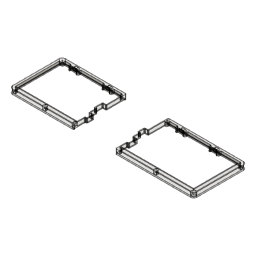
KBO-5000-Case-Redesign-Body (Autodesk Fusion 360 design; units mm, degrees)
Autodesk Fusion 360 part; units mm, degrees
(part 1 of 2)
other "Base Mesh Feature1"
sketch "Left-Main" plane through (0, 0, 0) normal (0, 0, 1) x (1, 0, 0)
  line L0 (-242, 0) -> (-78.0749, 0)
  line L1 (-250, 8) -> (-250, 135.063)
  line L2 (-242, 143.063) -> (-78.075, 143.063)
  line L3 (-76.075, 141.063) -> (-76.075, 90.2)
  line L4 (-78.075, 88.2) -> (-83.6, 88.2)
  line L5 (-85.6, 86.2) -> (-85.6, 71.15)
  line L6 (-83.6, 69.15) -> (-82.837, 69.15)
  line L7 (-80.837, 67.15) -> (-80.837, 52.1)
  line L8 (-78.837, 50.1) -> (-73.312, 50.1)
  line L9 (-71.312, 48.1) -> (-71.312, 33.05)
  line L10 (-73.312, 31.05) -> (-74.0741, 31.05)
  line L11 (-76.0741, 29.0501) -> (-76.0749, 1.9999)
  arc A0 (-242, 143.063) -> (-250, 135.063) centre (-242, 135.063) ccw
  arc A1 (-250, 8) -> (-242, 0) centre (-242, 8) ccw
  line L12 (-78.074, 32.05) -> (-78.0749, 2)
  line L13 (-242, 2) -> (-78.0749, 2)
  arc A2 (-248, 8) -> (-242, 2) centre (-242, 8) ccw
  line L14 (-248, 8) -> (-248, 135.063)
  arc A3 (-242, 141.063) -> (-248, 135.063) centre (-242, 135.063) ccw
  line L15 (-242, 141.063) -> (-78.075, 141.063)
  line L16 (-78.075, 141.063) -> (-78.075, 91.2)
  line L17 (-79.075, 90.2) -> (-86.6, 90.2)
  line L18 (-87.6, 89.2) -> (-87.6, 68.15)
  line L19 (-86.6, 67.15) -> (-83.837, 67.15)
  line L20 (-82.837, 66.15) -> (-82.837, 49.1)
  line L21 (-81.837, 48.1) -> (-74.312, 48.1)
  line L22 (-73.312, 47.1) -> (-73.312, 34.05)
  line L23 (-74.312, 33.05) -> (-77.074, 33.05)
  line L24 (-238.001, 131.063) -> (-237.9999, 12.005)
  line L25 (-78.075, 141.063) -> (-78.075, 131.063)
  arc A4 (-76.075, 141.063) -> (-78.075, 143.063) centre (-78.075, 141.063) ccw
  arc A5 (-78.0749, 0) -> (-76.0749, 1.9999) centre (-78.0749, 2) ccw
  arc A6 (-73.312, 31.05) -> (-71.312, 33.05) centre (-73.312, 33.05) ccw
  arc A7 (-71.312, 48.1) -> (-73.312, 50.1) centre (-73.312, 48.1) ccw
  arc A8 (-80.837, 52.1) -> (-78.837, 50.1) centre (-78.837, 52.1) ccw
  arc A9 (-80.837, 67.15) -> (-82.837, 69.15) centre (-82.837, 67.15) ccw
  arc A10 (-85.6, 71.15) -> (-83.6, 69.15) centre (-83.6, 71.15) ccw
  arc A11 (-83.6, 88.2) -> (-85.6, 86.2) centre (-83.6, 86.2) ccw
  arc A12 (-78.075, 88.2) -> (-76.075, 90.2) centre (-78.075, 90.2) ccw
  arc A13 (-79.075, 90.2) -> (-78.075, 91.2) centre (-79.075, 91.2) ccw
  arc A14 (-86.6, 90.2) -> (-87.6, 89.2) centre (-86.6, 89.2) ccw
  arc A15 (-87.6, 68.15) -> (-86.6, 67.15) centre (-86.6, 68.15) ccw
  arc A16 (-82.837, 66.15) -> (-83.837, 67.15) centre (-83.837, 66.15) ccw
  arc A17 (-82.837, 49.1) -> (-81.837, 48.1) centre (-81.837, 49.1) ccw
  arc A18 (-73.312, 47.1) -> (-74.312, 48.1) centre (-74.312, 47.1) ccw
  arc A19 (-74.312, 33.05) -> (-73.312, 34.05) centre (-74.312, 34.05) ccw
  arc A20 (-77.074, 33.05) -> (-78.074, 32.05) centre (-77.074, 32.05) ccw
  arc A21 (-74.0741, 31.05) -> (-76.0741, 29.0501) centre (-74.0741, 29.05) ccw
  line L26 (-237.9999, 12.005) -> (-78.0746, 11.9998)
  line L27 (-238.001, 131.063) -> (-78.075, 131.063)
  point P0 (-250, 0)
  point P1 (-76.075, 0)
  point P2 (-250, 143.063)
  point P3 (-76.075, 143.063)
  point P4 (-76.075, 88.2)
  point P5 (-85.6, 88.2)
  point P6 (-85.6, 69.15)
  point P7 (-80.837, 69.15)
  point P8 (-80.837, 50.1)
  point P9 (-71.312, 50.1)
  point P10 (-71.312, 31.05)
  point P11 (-76.074, 31.05)
  point P12 (-78.075, 131.063)
  dimension "d1" = 173.925
  dimension "d2" = 143.063
  dimension "d3" = 173.925
  dimension "d4" = 54.863
  dimension "d5" = 9.525
  dimension "d6" = 19.05
  dimension "d7" = 4.763
  dimension "d8" = 19.05
  dimension "d9" = 9.525
  dimension "d10" = 19.05
  dimension "d11" = 4.762
  dimension "d12" = 31.05
  dimension "d13" = 8
  dimension "d14" = 8
  dimension "d31" = 10
  dimension "d34" = 2
  dimension "d35" = 2
  dimension "d36" = 2
  dimension "d37" = 2
  dimension "d38" = 2
  dimension "d39" = 2
  dimension "d40" = 2
  dimension "d41" = 2
  dimension "d42" = 2
  dimension "d43" = 1
  dimension "d44" = 2
  dimension "d82" = 119.058
  constraint horizontal L0
  constraint perpendicular L0 L1
  constraint perpendicular L1 L2
  constraint perpendicular L2 L3
  constraint perpendicular L3 L4
  constraint perpendicular L4 L5
  constraint perpendicular L5 L6
  constraint perpendicular L6 L7
  constraint perpendicular L7 L8
  constraint perpendicular L8 L9
  constraint perpendicular L9 L10
  constraint coincident P2 L1
  constraint coincident P2 L2
  constraint tangent L1 A0
  constraint tangent L2 A0
  constraint coincident P0 L0
  constraint coincident P0 L1
  constraint tangent L0 A1
  constraint tangent L1 A1
  constraint concentric A1 A2
  constraint concentric A0 A3
  constraint tangent A3 L15
  constraint tangent L13 A2
  constraint tangent A2 L14
  constraint tangent L14 A3
  constraint coincident P12 L25.end
  constraint coincident P3 L2
  constraint coincident P3 L3
  constraint tangent L2 A4
  constraint tangent L3 A4
  constraint coincident P1 L0
  constraint coincident P1 L11
  constraint tangent L0 A5
  constraint tangent L11 A5
  constraint coincident P10 L9
  constraint coincident P10 L10
  constraint tangent L9 A6
  constraint tangent L10 A6
  constraint coincident P9 L8
  constraint coincident P9 L9
  constraint tangent L8 A7
  constraint tangent L9 A7
  constraint coincident P8 L7
  constraint coincident P8 L8
  constraint tangent L7 A8
  constraint tangent L8 A8
  constraint coincident P7 L6
  constraint coincident P7 L7
  constraint tangent L6 A9
  constraint tangent L7 A9
  constraint coincident P6 L5
  constraint coincident P6 L6
  constraint tangent L5 A10
  constraint tangent L6 A10
  constraint coincident P5 L4
  constraint coincident P5 L5
  constraint tangent L4 A11
  constraint tangent L5 A11
  constraint coincident P4 L3
  constraint coincident P4 L4
  constraint tangent L3 A12
  constraint tangent L4 A12
  constraint tangent L16 A13
  constraint tangent L17 A13
  constraint tangent L17 A14
  constraint tangent L18 A14
  constraint equal A13 A14
  constraint tangent L18 A15
  constraint tangent L19 A15
  constraint equal A13 A15
  constraint tangent L19 A16
  constraint tangent L20 A16
  constraint equal A13 A16
  constraint tangent L20 A17
  constraint tangent L21 A17
  constraint equal A13 A17
  constraint tangent L21 A18
  constraint tangent L22 A18
  constraint equal A13 A18
  constraint tangent L22 A19
  constraint tangent L23 A19
  constraint equal A13 A19
  constraint tangent L12 A20
  constraint tangent L23 A20
  constraint equal A13 A20
  constraint coincident P11 L10
  constraint coincident P11 L11
  constraint tangent L10 A21
  constraint tangent L11 A21
  constraint coincident L12 L26.end
  constraint perpendicular L12 L26
  constraint perpendicular L25 L27
  measures "d1" distance of P0 P1
  measures "d2" distance of P0 P2
  measures "d3" distance of P2 P3
  measures "d4" distance of P3 P4
  measures "d5" distance of P4 P5
  measures "d6" distance of P5 P6
  measures "d7" distance of P6 P7
  measures "d8" distance of P7 P8
  measures "d9" distance of P8 P9
  measures "d10" distance of P9 P10
  measures "d11" distance of P10 P11
  measures "d12" distance of L0 L10
  measures "d13" radius of A0
  measures "d14" radius of A1
  measures "d31" distance of L15.end P12
  measures "d34" radius of A4
  measures "d35" radius of A5
  measures "d36" radius of A6
  measures "d37" radius of A7
  measures "d38" radius of A8
  measures "d39" radius of A9
  measures "d40" radius of A10
  measures "d41" radius of A11
  measures "d42" radius of A12
  measures "d43" radius of A13
  measures "d44" radius of A21
  measures "d82" vertical distance of L24.start L24.end
sketch "Left-Bottom" plane through (0, 0, 0) normal (0, 0, 1) x (1, 0, 0)
  line L0 (-76.0749, 3.75) -> (-76.0749, 1.9999)
  line L1 (-78.0749, 0) -> (-242, 0)
  line L2 (-76.0749, 3.75) -> (-242, 3.7553)
  line L3 (-78.075, 143.063) -> (-242, 143.063)
  line L4 (-76.075, 141.063) -> (-76.075, 139.313)
  line L5 (-76.075, 139.313) -> (-242, 139.313)
  line L6 (-250, 135.063) -> (-250, 8)
  line L7 (-246.25, 135.063) -> (-246.2499, 8.0053)
  arc A0 (-250, 8) -> (-242, 0) centre (-242, 8) ccw
  arc A1 (-242, 143.063) -> (-250, 135.063) centre (-242, 135.063) ccw
  arc A2 (-242, 139.313) -> (-246.25, 135.063) centre (-242, 135.063) ccw
  arc A3 (-246.2499, 8.0053) -> (-242, 3.7553) centre (-241.9999, 8.0053) ccw
  arc A4 (-76.075, 141.063) -> (-78.075, 143.063) centre (-78.075, 141.063) ccw
  arc A5 (-78.0749, 0) -> (-76.0749, 1.9999) centre (-78.0749, 2) ccw
  circle A6 centre (-80.0748, 135.0624) radius 2.9
  circle A7 centre (-80.0748, 135.0624) radius 1.2
  circle A8 centre (-80.0749, 8) radius 2.9
  circle A9 centre (-80.0749, 8) radius 1.2
  circle A10 centre (-108.9375, 135.0625) radius 1.2
  circle A11 centre (-128.9375, 135.0625) radius 1.2
  circle A12 centre (-199.425, 135.0625) radius 1.2
  circle A13 centre (-219.425, 135.0625) radius 1.2
  circle A14 centre (-241.4142, 134.4767) radius 1.2
  circle A15 centre (-241.4142, 8.5857) radius 1.2
  circle A16 centre (-160.0375, 8) radius 1.2
  circle A17 centre (-241.4142, 134.4767) radius 2.9
  circle A18 centre (-241.4142, 8.5857) radius 2.9
  circle A19 centre (-160.0375, 8) radius 2.9
  line L8 (-126.938, 132.063) -> (-126.938, 133.063)
  line L9 (-125.938, 134.063) -> (-111.938, 134.063)
  line L10 (-110.938, 133.063) -> (-110.938, 132.063)
  arc A20 (-125.938, 134.063) -> (-126.938, 133.063) centre (-125.938, 133.063) ccw
  arc A21 (-110.938, 133.063) -> (-111.938, 134.063) centre (-111.938, 133.063) ccw
  line L11 (-109.938, 131.063) -> (-108.938, 131.063)
  line L12 (-127.938, 131.063) -> (-128.938, 131.063)
  arc A22 (-110.938, 132.063) -> (-109.938, 131.063) centre (-109.938, 132.063) ccw
  arc A23 (-127.938, 131.063) -> (-126.938, 132.063) centre (-127.938, 132.063) ccw
  line L13 (-128.938, 131.063) -> (-128.938, 130.063)
  line L14 (-128.938, 130.063) -> (-108.938, 130.063)
  line L15 (-108.938, 130.063) -> (-108.938, 131.063)
  line L16 (-216.425, 134.063) -> (-202.425, 134.063)
  line L17 (-201.425, 133.063) -> (-201.425, 132.063)
  line L18 (-217.425, 132.063) -> (-217.425, 133.063)
  line L19 (-200.425, 131.063) -> (-199.425, 131.063)
  line L20 (-199.425, 131.063) -> (-199.425, 130.063)
  line L21 (-199.425, 130.063) -> (-201.425, 130.063)
  line L22 (-218.425, 131.063) -> (-219.425, 131.063)
  line L23 (-219.425, 131.063) -> (-219.425, 130.063)
  line L24 (-219.425, 130.063) -> (-217.425, 130.063)
  line L25 (-201.425, 130.063) -> (-217.425, 130.063)
  arc A24 (-201.425, 133.063) -> (-202.425, 134.063) centre (-202.425, 133.063) ccw
  arc A25 (-216.425, 134.063) -> (-217.425, 133.063) centre (-216.425, 133.063) ccw
  arc A26 (-218.425, 131.063) -> (-217.425, 132.063) centre (-218.425, 132.063) ccw
  arc A27 (-201.425, 132.063) -> (-200.425, 131.063) centre (-200.425, 132.063) ccw
  circle A28 centre (-108.9375, 135.0625) radius 2.9
  circle A29 centre (-128.9375, 135.0625) radius 2.9
  circle A30 centre (-199.425, 135.0625) radius 2.9
  circle A31 centre (-219.425, 135.0625) radius 2.9
  point P0 (-76.0749, 3.75)
  point P1 (-76.075, 0)
  point P2 (-246.2499, 3.7554)
  point P3 (-76.075, 143.063)
  point P4 (-246.25, 139.313)
  point P5 (-110.938, 131.063)
  point P6 (-126.938, 131.063)
  point P7 (-110.938, 134.063)
  point P8 (-217.425, 134.063)
  point P9 (-217.425, 134.063)
  point P10 (-201.425, 134.063)
  point P11 (-201.425, 131.063)
  point P12 (-217.425, 131.063)
  dimension "d51" = 170.175
  dimension "d52" = 3.75
  dimension "d53" = 3.75
  dimension "d54" = 170.175
  dimension "d55" = 8
  dimension "d56" = 8
  dimension "d57" = 4.25
  dimension "d58" = 4.25
  dimension "d62" = 2
  dimension "d63" = 2
  dimension "d64" = 2.4
  dimension "d65" = 5.8
  dimension "d66" = 2.4
  dimension "d67" = 5.8
  dimension "d68" = 2.4
  dimension "d70" = 2.4
  dimension "d72" = 2.4
  dimension "d75" = 2.4
  dimension "d76" = 2.4
  dimension "d77" = 5.8
  dimension "d78" = 2.4
  dimension "d79" = 5.8
  dimension "d80" = 2.4
  dimension "d81" = 5.8
  dimension "d86" = 16
  dimension "d87" = 3
  dimension "d88" = 1
  dimension "d89" = 2
  dimension "d90" = 2
  dimension "d91" = 1
  dimension "d92" = 1
  dimension "d93" = 20
  dimension "d94" = 1
  dimension "d99" = 16
  dimension "d100" = 3
  dimension "d101" = 2
  dimension "d102" = 1
  dimension "d103" = 2
  dimension "d104" = 1
  dimension "d105" = 1
  dimension "d154" = 5.8
  dimension "d155" = 5.8
  dimension "d156" = 5.8
  dimension "d157" = 5.8
  constraint coincident P0 L0.start
  constraint perpendicular L0 L2
  constraint perpendicular L3 L4
  constraint perpendicular L4 L5
  constraint tangent L6 A0
  constraint tangent L1 A0
  constraint tangent L6 A1
  constraint tangent L3 A1
  constraint coincident P4 L5
  constraint coincident P4 L7
  constraint tangent L5 A2
  constraint tangent L7 A2
  constraint coincident P2 L2
  constraint coincident P2 L7
  constraint tangent L2 A3
  constraint tangent L7 A3
  constraint tangent L4 A4
  constraint tangent L3 A4
  constraint tangent L0 A5
  constraint tangent L1 A5
  constraint concentric A6 A7
  constraint concentric A8 A9
  constraint concentric A14 A17
  constraint concentric A15 A18
  constraint concentric A16 A19
  constraint vertical L8
  constraint horizontal L9
  constraint vertical L10
  constraint tangent L8 A20
  constraint tangent L9 A20
  constraint coincident P7 L9
  constraint coincident P7 L10
  constraint tangent L9 A21
  constraint tangent L10 A21
  constraint equal A20 A21
  constraint perpendicular L10 L11
  constraint perpendicular L8 L12
  constraint coincident P5 L10
  constraint coincident P5 L11
  constraint tangent L10 A22
  constraint tangent L11 A22
  constraint coincident P6 L8
  constraint coincident P6 L12
  constraint tangent L8 A23
  constraint tangent L12 A23
  constraint vertical L13
  constraint horizontal L14
  constraint vertical L15
  constraint horizontal L16
  constraint vertical L17
  constraint vertical L18
  constraint coincident P9 P8
  constraint horizontal L19
  constraint vertical L20
  constraint horizontal L21
  constraint horizontal L22
  constraint vertical L23
  constraint horizontal L24
  constraint horizontal L25
  constraint coincident P10 L16
  constraint coincident P10 L17
  constraint tangent L16 A24
  constraint tangent L17 A24
  constraint coincident P9 L16
  constraint coincident P9 L18
  constraint tangent L16 A25
  constraint tangent L18 A25
  constraint equal A24 A25
  constraint coincident P12 L18
  constraint coincident P12 L22
  constraint tangent L18 A26
  constraint tangent L22 A26
  constraint equal A24 A26
  constraint coincident P11 L17
  constraint coincident P11 L19
  constraint tangent L17 A27
  constraint tangent L19 A27
  constraint equal A24 A27
  constraint concentric A10 A28
  constraint concentric A11 A29
  constraint concentric A12 A30
  constraint concentric A13 A31
  measures "d51" distance of P0 P2
  measures "d52" vertical distance of P1 P0
  measures "d53" distance of P3 L4.end
  measures "d54" distance of L4.end P4
  measures "d55" radius of A0
  measures "d56" radius of A1
  measures "d57" radius of A2
  measures "d58" radius of A3
  measures "d62" radius of A4
  measures "d63" radius of A5
  measures "d64" diameter of A7
  measures "d65" diameter of A6
  measures "d66" diameter of A9
  measures "d67" diameter of A8
  measures "d68" diameter of A10
  measures "d70" diameter of A11
  measures "d72" diameter of A12
  measures "d75" diameter of A13
  measures "d76" diameter of A14
  measures "d77" diameter of A17
  measures "d78" diameter of A15
  measures "d79" diameter of A18
  measures "d80" diameter of A16
  measures "d81" diameter of A19
  measures "d86" distance of P5 P6
  measures "d87" distance of P5 P7
  measures "d88" radius of A20
  measures "d89" distance of P5 L11.end
  measures "d90" distance of P6 L12.end
  measures "d91" radius of A22
  measures "d92" radius of A23
  measures "d93" distance of L11.end L12.end
  measures "d94" distance of L11.end L14.end
  measures "d99" distance of P9 P10
  measures "d100" distance of P9 P12
  measures "d101" distance of P11 L19.end
  measures "d102" distance of P11 L21.end
  measures "d103" distance of P12 L22.end
  measures "d104" distance of P12 L24.end
  measures "d105" radius of A24
  measures "d154" diameter of A28
  measures "d155" diameter of A29
  measures "d156" diameter of A30
  measures "d157" diameter of A31
sketch "Left-USB" plane through (0, 0, 0) normal (0, 1, 0) x (1, 0, 0)
  line L0 (-121.8375, -8) -> (-116.0375, -8)
  arc A0 (-116.0375, -8) -> (-116.0375, -4.2) centre (-116.0375, -6.1) ccw
  line L1 (-116.0375, -4.2) -> (-121.8375, -4.2)
  arc A1 (-121.8375, -4.2) -> (-121.8375, -8) centre (-121.8375, -6.1) ccw
  arc A2 (-116.0375, -10.1) -> (-116.0375, -2.1) centre (-116.0375, -6.1) ccw
  line L2 (-116.0375, -2.1) -> (-121.8375, -2.1)
  arc A3 (-121.8375, -2.1) -> (-121.8375, -10.1) centre (-121.8375, -6.1) ccw
  line L3 (-121.8375, -10.1) -> (-116.0375, -10.1)
  arc A4 (-116.0375, -12) -> (-112.1069, -1.7) centre (-116.0375, -6.1) ccw
  arc A5 (-125.7682, -1.7) -> (-121.8375, -12) centre (-121.8375, -6.1) ccw
  line L4 (-121.8375, -12) -> (-116.0375, -12)
  arc A6 (-206.525, -8) -> (-206.525, -4.2) centre (-206.525, -6.1) ccw
  line L5 (-206.525, -4.2) -> (-212.325, -4.2)
  arc A7 (-212.325, -4.2) -> (-212.325, -8) centre (-212.325, -6.1) ccw
  line L6 (-212.325, -8) -> (-206.525, -8)
  arc A8 (-206.525, -10.1) -> (-206.525, -2.1) centre (-206.525, -6.1) ccw
  line L7 (-206.525, -2.1) -> (-212.325, -2.1)
  arc A9 (-212.325, -2.1) -> (-212.325, -10.1) centre (-212.325, -6.1) ccw
  line L8 (-212.325, -10.1) -> (-206.525, -10.1)
  arc A10 (-206.525, -12) -> (-202.5944, -1.7) centre (-206.525, -6.1) ccw
  arc A11 (-216.2557, -1.7) -> (-212.325, -12) centre (-212.325, -6.1) ccw
  line L9 (-212.325, -12) -> (-206.525, -12)
  line L10 (-114.1375, -6.1) -> (-114.1375, -7.4)
  line L11 (-114.1375, -7.4) -> (-113.3875, -7.4)
  line L12 (-113.3875, -7.4) -> (-113.3875, -11.3)
  line L13 (-114.1375, -6.1) -> (-123.7375, -6.1)
  line L14 (-123.7375, -6.1) -> (-123.7375, -7.4)
  line L15 (-114.1375, -7.4) -> (-114.1375, -6.1)
  line L16 (-124.4875, -7.4) -> (-124.4875, -11.3)
  line L17 (-124.4875, -11.3) -> (-113.3875, -11.3)
  line L18 (-113.3875, -11.3) -> (-113.3875, -7.4)
  line L19 (-113.3875, -7.4) -> (-114.1375, -7.4)
  line L20 (-123.7375, -7.4) -> (-124.4875, -7.4)
  line L21 (-206.525, -6.1) -> (-204.625, -6.1)
  line L22 (-204.625, -6.1) -> (-204.625, -7.4)
  line L23 (-204.625, -7.4) -> (-203.875, -7.4)
  line L24 (-203.875, -7.4) -> (-203.875, -11.3)
  line L25 (-204.625, -6.1) -> (-214.225, -6.1)
  line L26 (-214.225, -6.1) -> (-214.225, -7.4)
  line L27 (-204.625, -7.4) -> (-204.625, -6.1)
  line L28 (-214.975, -7.4) -> (-214.975, -11.3)
  line L29 (-214.975, -11.3) -> (-203.875, -11.3)
  line L30 (-203.875, -11.3) -> (-203.875, -7.4)
  line L31 (-203.875, -7.4) -> (-204.625, -7.4)
  line L32 (-214.225, -7.4) -> (-214.975, -7.4)
  line L33 (-112.1069, -1.7) -> (-125.7682, -1.7)
  line L34 (-202.5944, -1.7) -> (-216.2557, -1.7)
  dimension "d118" = 2.1
  dimension "d122" = 2.1
  dimension "d124" = 1.9
  dimension "d125" = 1.3
  dimension "d126" = 0.75
  dimension "d127" = 3.9
  dimension "d128" = 9.6
  dimension "d130" = 11.1
  dimension "d132" = 1.9
  dimension "d134" = 0.75
  dimension "d136" = 9.6
  dimension "d137" = 1.3
  dimension "d138" = 11.1
  dimension "d139" = 3.9
  constraint tangent L0 A0
  constraint tangent L1 A1
  constraint tangent A6 L6
  constraint tangent A6 L5
  constraint tangent L5 A7
  constraint tangent A7 L6
  constraint perpendicular L10 L11
  constraint perpendicular L11 L12
  constraint horizontal L13
  constraint vertical L14
  constraint vertical L15
  constraint horizontal L19
  constraint vertical L16
  constraint horizontal L17
  constraint vertical L18
  constraint collinear L19 L20
  constraint coincident A6.centre A8.centre
  constraint midpoint A6 L21.end
  constraint horizontal L21
  constraint perpendicular L21 L22
  constraint perpendicular L22 L23
  constraint perpendicular L23 L24
  constraint horizontal L25
  constraint vertical L26
  constraint vertical L27
  constraint horizontal L31
  constraint vertical L28
  constraint horizontal L29
  constraint vertical L30
  constraint collinear L31 L32
  constraint concentric A0 A4
  constraint concentric A1 A5
  constraint tangent A4 L4
  constraint tangent A5 L4
  constraint concentric A6 A10
  constraint concentric A7 A11
  constraint tangent A11 L9
  constraint tangent A10 L9
  measures "d124" distance of A0.centre L10.start
  measures "d125" distance of L10.start L10.end
  measures "d126" distance of L10.end L11.end
  measures "d127" distance of L11.end L12.end
  measures "d128" distance of L10.start L13.end
  measures "d130" distance of L11.end L16.start
  measures "d132" distance of A6.centre L21.end
  measures "d134" distance of L22.end L23.end
  measures "d136" distance of L21.end L25.end
  measures "d137" distance of L21.end L22.end
  measures "d138" distance of L23.end L28.start
  measures "d139" distance of L23.end L24.end
sketch "Left-Holders" plane through (0, 0, 0) normal (0, 0, 1) x (1, 0, 0)
  line L0 (-76.075, 141.063) -> (-76.075, 131.063)
  line L1 (-76.075, 131.063) -> (-80.075, 131.063)
  line L2 (-84.075, 135.063) -> (-84.075, 143.063)
  line L3 (-84.075, 143.063) -> (-78.075, 143.063)
  line L4 (-78.075, 143.063) -> (-76.075, 141.063)
  arc A0 (-84.075, 135.063) -> (-80.075, 131.063) centre (-80.075, 135.063) ccw
  line L5 (-241, 143.063) -> (-238, 143.063)
  line L6 (-238, 143.063) -> (-238, 135.063)
  line L7 (-242, 131.063) -> (-250, 131.063)
  line L8 (-250, 131.063) -> (-250, 134.063)
  arc A1 (-241, 143.063) -> (-250, 134.063) centre (-241, 134.063) ccw
  arc A2 (-242, 131.063) -> (-238, 135.063) centre (-242, 135.063) ccw
  line L9 (-241, 0) -> (-238, 0)
  line L10 (-238, 0) -> (-238, 8)
  line L11 (-242, 12) -> (-250, 12)
  line L12 (-250, 12) -> (-250, 9)
  arc A3 (-250, 9) -> (-241, 0) centre (-241, 9) ccw
  arc A4 (-238, 8) -> (-242, 12) centre (-242, 8) ccw
  line L13 (-79.075, 0) -> (-84.075, 0)
  line L14 (-84.075, 0) -> (-84.075, 8)
  line L15 (-80.075, 12) -> (-76.075, 12)
  line L16 (-76.075, 12) -> (-76.075, 3)
  arc A5 (-79.075, 0) -> (-76.075, 3) centre (-79.075, 3) ccw
  arc A6 (-80.075, 12) -> (-84.075, 8) centre (-80.075, 8) ccw
  line L17 (-156.0375, 0) -> (-164.0375, 0)
  line L18 (-164.0375, 0) -> (-164.0375, 8)
  line L19 (-156.0375, 8) -> (-156.0375, 0)
  arc A7 (-156.0375, 8) -> (-160.0375, 12) centre (-160.0375, 8) ccw
  arc A8 (-160.0375, 12) -> (-164.0375, 8) centre (-160.0375, 8) ccw
  line L20 (-104.9375, 143.063) -> (-132.9375, 143.063)
  line L21 (-132.9375, 143.063) -> (-132.9375, 135.063)
  line L22 (-128.9375, 131.063) -> (-108.9375, 131.063)
  line L23 (-104.9375, 135.063) -> (-104.9375, 143.063)
  arc A9 (-108.9375, 131.063) -> (-104.9375, 135.063) centre (-108.9375, 135.063) ccw
  arc A10 (-132.9375, 135.063) -> (-128.9375, 131.063) centre (-128.9375, 135.063) ccw
  line L24 (-195.425, 143.063) -> (-223.425, 143.063)
  line L25 (-223.425, 143.063) -> (-223.425, 135.063)
  line L26 (-219.425, 131.063) -> (-199.425, 131.063)
  line L27 (-195.425, 135.063) -> (-195.425, 143.063)
  arc A11 (-199.425, 131.063) -> (-195.425, 135.063) centre (-199.425, 135.063) ccw
  arc A12 (-223.425, 135.063) -> (-219.425, 131.063) centre (-219.425, 135.063) ccw
  point P0 (-84.075, 131.063)
  point P1 (-156.0375, 12)
  point P2 (-108.9375, 135.0625)
  point P3 (-104.9375, 131.063)
  point P4 (-195.425, 131.063)
  dimension "d164" = 10
  dimension "d165" = 8
  dimension "d169" = 4
  dimension "d172" = 9
  dimension "d173" = 4
  dimension "d176" = 9
  dimension "d177" = 4
  dimension "d180" = 3
  dimension "d181" = 4
  dimension "d183" = 8
  dimension "d184" = 12
  dimension "d185" = 4
  dimension "d186" = 4
  dimension "d188" = 28
  dimension "d189" = 12
  dimension "d190" = 4
  dimension "d193" = 28
  dimension "d194" = 12
  dimension "d195" = 4
  constraint horizontal L1
  constraint vertical L2
  constraint horizontal L3
  constraint coincident P0 L1
  constraint coincident P0 L2
  constraint tangent L1 A0
  constraint tangent L2 A0
  constraint horizontal L5
  constraint vertical L6
  constraint horizontal L7
  constraint vertical L8
  constraint tangent L5 A1
  constraint tangent L8 A1
  constraint tangent L6 A2
  constraint tangent L7 A2
  constraint horizontal L9
  constraint vertical L10
  constraint horizontal L11
  constraint vertical L12
  constraint tangent L9 A3
  constraint tangent L12 A3
  constraint tangent L10 A4
  constraint tangent L11 A4
  constraint horizontal L13
  constraint vertical L14
  constraint horizontal L15
  constraint vertical L16
  constraint tangent L13 A5
  constraint tangent L16 A5
  constraint tangent L14 A6
  constraint tangent L15 A6
  constraint horizontal L17
  constraint vertical L18
  constraint vertical L19
  constraint coincident P1 L19
  constraint tangent L19 A7
  constraint tangent L18 A8
  constraint coincident A7.end A8.start
  constraint horizontal L20
  constraint vertical L21
  constraint horizontal L22
  constraint vertical L23
  constraint coincident P3 L22
  constraint coincident P3 L23
  constraint tangent L22 A9
  constraint tangent L23 A9
  constraint tangent L21 A10
  constraint tangent L22 A10
  constraint equal A9 A10
  constraint horizontal L24
  constraint vertical L25
  constraint horizontal L26
  constraint vertical L27
  constraint coincident P4 L26
  constraint coincident P4 L27
  constraint tangent L26 A11
  constraint tangent L27 A11
  constraint tangent L25 A12
  constraint tangent L26 A12
  constraint equal A11 A12
  measures "d164" distance of L0.start L0.end
  measures "d165" distance of L0.end P0
  measures "d169" radius of A0
  measures "d172" radius of A1
  measures "d173" radius of A2
  measures "d176" radius of A3
  measures "d177" radius of A4
  measures "d180" radius of A5
  measures "d181" radius of A6
  measures "d183" distance of L17.start L17.end
  measures "d184" distance of L17.start P1
  measures "d185" radius of A7
  measures "d186" radius of A8
  measures "d188" distance of L20.start L20.end
  measures "d189" distance of L20.start P3
  measures "d190" radius of A9
  measures "d193" distance of L24.start L24.end
  measures "d194" distance of L24.start P4
  measures "d195" radius of A11
extrude "Extrude-Side" add sketch "Left-Main" along normal blind 11 from surface at 1.7 makes body 1
extrude "Extrude-Top" add sketch "Left-Main" along normal blind 1.8 from surface at 10.9 contours L12 L13 A2 L14 A3 L15 L16 L24 L25 L26 L27 bodies 1
extrude "Extrude-Side2" add sketch "Left-Bottom" along normal blind 11 contours L0 L1 L2 L3 L4 L5 L6 L7 A0 A1 A2 A3 A4 A5 bodies 1
extrude "Extrude-Holder" add sketch "Left-Bottom" along normal blind 11 from surface at 1.7 contours A6 | A8 | A17 | A18 | A19 | L8 A20 A29 | L8 A20 A29 | L10 A21 A28 | L10 A21 A28 | L18 A25 A31 | L18 A25 A31 | L17 A24 A30 | L17 A24 A30 bodies 1
extrude "Extrude-Holder-2" add sketch "Left-Holders" along normal blind 9.3 from surface at 1.7 bodies 1
extrude "Cut-USB-Out" cut sketch "Left-USB" along normal blind 15 from surface at 137.043 contours L0 A0 A1 L13 | L0 A0 A1 A2 A3 L3 L10 L11 L12 L14 L15 L16 L18 L19 L20 | A0 L1 A1 A2 L2 A3 L10 L11 L12 L14 L15 L16 L18 L19 L20 | A0 L1 A1 L13 | A6 A7 L6 L21 L25 | A6 A7 L6 A8 A9 L8 L22 L23 L24 L26 L27 L28 L30 L31 L32 | A6 L5 A7 L21 L25 | A6 L5 A7 A8 L7 A9 L22 L23 L24 L26 L27 L28 L30 L31 L32 bodies 1
extrude "Cut-USB-In" cut sketch "Left-USB" along normal blind 3.5 from surface at 132.063 contours L0 A0 A1 L13 | L0 A0 A1 A2 A3 L3 L10 L11 L12 L14 L15 L16 L18 L19 L20 | A2 A3 L3 L12 L16 L17 L18 | A6 A7 L6 L21 L25 | A6 A7 L6 A8 A9 L8 L22 L23 L24 L26 L27 L28 L30 L31 L32 | A8 A9 L8 L24 L28 L29 L30 bodies 1
extrude "Cut-USB-In-2" cut sketch "Left-Bottom" along normal blind 13 contours L8 L9 L10 A20 A21 L11 L12 A22 A23 L13 L14 L15 A28 A29 | L8 A20 A29 | L10 A21 A28 | L16 L17 L18 L19 L20 L21 L22 L23 L24 L25 A24 A25 A26 A27 A30 A31 | L18 A25 A31 | L17 A24 A30 picked at (-126.616, 133.5034) picked at (-111.2595, 133.5035) picked at (-217.1033, 133.5035) picked at (-201.7468, 133.5035) bodies 1
extrude "Cut-Screw-Holes" cut sketch "Left-Bottom" along normal blind 15 contours A7 | A9 | A10 | A11 | A12 | A13 | A14 | A15 | A16 bodies 1
extrude "Cut-USB-through" cut sketch "Left-USB" along normal blind 20 from surface at 130 contours L0 A0 A1 L13 | A0 L1 A1 L13 | A6 A7 L6 L21 L25 | A6 L5 A7 L21 L25 bodies 1
sketch "Right-Main" plane through (0, 0, 0) normal (0, 0, 1) x (1, 0, 0)
  line L0 (242, 0) -> (39.975, 0)
  line L1 (250, 8) -> (250, 135.062)
  line L2 (242, 143.062) -> (39.975, 143.062)
  line L3 (37.975, 141.062) -> (37.975, 90.199)
  line L4 (35.975, 88.199) -> (30.45, 88.199)
  line L5 (28.45, 86.199) -> (28.45, 71.149)
  line L6 (30.45, 69.149) -> (31.212, 69.149)
  line L7 (33.212, 67.149) -> (33.212, 52.099)
  line L8 (35.212, 50.099) -> (40.737, 50.099)
  line L9 (42.737, 48.099) -> (42.737, 33.049)
  line L10 (40.737, 31.049) -> (39.975, 31.049)
  line L11 (37.975, 29.049) -> (37.975, 2)
  line L12 (238, 12) -> (238, 131.063)
  line L13 (238, 131.063) -> (39.975, 131.063)
  line L14 (238, 12) -> (39.975, 12)
  line L15 (39.975, 143.062) -> (39.975, 87.199)
  line L16 (38.975, 86.199) -> (31.45, 86.199)
  line L17 (30.45, 85.199) -> (30.45, 72.149)
  line L18 (31.45, 71.149) -> (34.212, 71.149)
  line L19 (35.212, 70.149) -> (35.212, 53.099)
  line L20 (36.212, 52.099) -> (43.737, 52.099)
  line L21 (44.737, 51.099) -> (44.737, 30.049)
  line L22 (43.737, 29.049) -> (40.975, 29.049)
  line L23 (39.975, 28.049) -> (39.975, 0)
  arc A0 (250, 135.062) -> (242, 143.062) centre (242, 135.062) ccw
  arc A1 (242, 0) -> (250, 8) centre (242, 8) ccw
  arc A2 (39.975, 143.062) -> (37.975, 141.062) centre (39.975, 141.062) ccw
  arc A3 (37.975, 2) -> (39.975, 0) centre (39.975, 2) ccw
  arc A4 (38.975, 86.199) -> (39.975, 87.199) centre (38.975, 87.199) ccw
  arc A5 (35.975, 88.199) -> (37.975, 90.199) centre (35.975, 90.199) ccw
  arc A6 (30.45, 88.199) -> (28.45, 86.199) centre (30.45, 86.199) ccw
  arc A7 (31.45, 86.199) -> (30.45, 85.199) centre (31.45, 85.199) ccw
  arc A8 (28.45, 71.149) -> (30.45, 69.149) centre (30.45, 71.149) ccw
  arc A9 (33.212, 67.149) -> (31.212, 69.149) centre (31.212, 67.149) ccw
  arc A10 (33.212, 52.099) -> (35.212, 50.099) centre (35.212, 52.099) ccw
  arc A11 (42.737, 48.099) -> (40.737, 50.099) centre (40.737, 48.099) ccw
  arc A12 (40.737, 31.049) -> (42.737, 33.049) centre (40.737, 33.049) ccw
  arc A13 (39.975, 31.049) -> (37.975, 29.049) centre (39.975, 29.049) ccw
  arc A14 (40.975, 29.049) -> (39.975, 28.049) centre (40.975, 28.049) ccw
  arc A15 (35.212, 70.149) -> (34.212, 71.149) centre (34.212, 70.149) ccw
  arc A16 (30.45, 72.149) -> (31.45, 71.149) centre (31.45, 72.149) ccw
  arc A17 (35.212, 53.099) -> (36.212, 52.099) centre (36.212, 53.099) ccw
  arc A18 (44.737, 51.099) -> (43.737, 52.099) centre (43.737, 51.099) ccw
  arc A19 (43.737, 29.049) -> (44.737, 30.049) centre (43.737, 30.049) ccw
  point P0 (250, 143.062)
  point P1 (37.975, 143.062)
  point P2 (37.975, 88.199)
  point P3 (28.45, 88.199)
  point P4 (28.45, 69.149)
  point P5 (33.212, 69.149)
  point P6 (33.212, 50.099)
  point P7 (42.737, 50.099)
  point P8 (42.737, 31.049)
  point P9 (37.975, 31.049)
  dimension "d206" = 212.025
  dimension "d207" = 54.863
  dimension "d208" = 9.525
  dimension "d209" = 19.05
  dimension "d210" = 4.762
  dimension "d211" = 19.05
  dimension "d212" = 9.525
  dimension "d213" = 19.05
  dimension "d214" = 4.762
  dimension "d217" = 119.063
  dimension "d218" = 198.025
  dimension "d219" = 198.025
  dimension "d221" = 8
  dimension "d222" = 8
  dimension "d227" = 2
  dimension "d228" = 2
  dimension "d229" = 1
  dimension "d230" = 2
  dimension "d231" = 2
  dimension "d232" = 1
  dimension "d233" = 2
  dimension "d234" = 2
  dimension "d235" = 2
  dimension "d236" = 2
  dimension "d237" = 2
  dimension "d238" = 2
  dimension "d239" = 1
  dimension "d240" = 1
  dimension "d241" = 1
  dimension "d242" = 1
  dimension "d243" = 1
  dimension "d244" = 1
  constraint horizontal L0
  constraint perpendicular L0 L1
  constraint perpendicular L1 L2
  constraint perpendicular L2 L3
  constraint perpendicular L3 L4
  constraint perpendicular L4 L5
  constraint perpendicular L5 L6
  constraint perpendicular L4 L7
  constraint perpendicular L7 L8
  constraint perpendicular L8 L9
  constraint perpendicular L9 L10
  constraint perpendicular L12 L13
  constraint perpendicular L12 L14
  constraint coincident P0 L1
  constraint coincident P0 L2
  constraint tangent L1 A0
  constraint tangent L2 A0
  constraint tangent L0 A1
  constraint tangent L1 A1
  constraint coincident P1 L2
  constraint coincident P1 L3
  constraint tangent L2 A2
  constraint tangent L3 A2
  constraint tangent L0 A3
  constraint tangent L11 A3
  constraint tangent L15 A4
  constraint tangent L16 A4
  constraint coincident P2 L3
  constraint coincident P2 L4
  constraint tangent L3 A5
  constraint tangent L4 A5
  constraint coincident P3 L4
  constraint coincident P3 L5
  constraint tangent L4 A6
  constraint tangent L5 A6
  constraint tangent L16 A7
  constraint tangent L17 A7
  constraint coincident P4 L5
  constraint coincident P4 L6
  constraint tangent L5 A8
  constraint tangent L6 A8
  constraint coincident P5 L6
  constraint coincident P5 L7
  constraint tangent L6 A9
  constraint tangent L7 A9
  constraint coincident P6 L7
  constraint coincident P6 L8
  constraint tangent L7 A10
  constraint tangent L8 A10
  constraint coincident P7 L8
  constraint coincident P7 L9
  constraint tangent L8 A11
  constraint tangent L9 A11
  constraint coincident P8 L9
  constraint coincident P8 L10
  constraint tangent L9 A12
  constraint tangent L10 A12
  constraint coincident P9 L10
  constraint coincident P9 L11
  constraint tangent L10 A13
  constraint tangent L11 A13
  constraint tangent L22 A14
  constraint tangent L23 A14
  constraint tangent L18 A15
  constraint tangent L19 A15
  constraint tangent L17 A16
  constraint tangent L18 A16
  constraint tangent L19 A17
  constraint tangent L20 A17
  constraint tangent L20 A18
  constraint tangent L21 A18
  constraint tangent L21 A19
  constraint tangent L22 A19
  measures "d206" distance of P0 P1
  measures "d207" distance of P1 P2
  measures "d208" distance of P2 P3
  measures "d209" distance of P3 P4
  measures "d210" distance of P4 P5
  measures "d211" distance of P5 P6
  measures "d212" distance of P6 P7
  measures "d213" distance of P7 P8
  measures "d214" distance of P8 P9
  measures "d217" distance of L12.start L12.end
  measures "d218" distance of L12.end L13.end
  measures "d219" distance of L12.start L14.end
  measures "d221" radius of A0
  measures "d222" radius of A1
  measures "d227" radius of A2
  measures "d228" radius of A3
  measures "d229" radius of A4
  measures "d230" radius of A5
  measures "d231" radius of A6
  measures "d232" radius of A7
  measures "d233" radius of A8
  measures "d234" radius of A9
  measures "d235" radius of A10
  measures "d236" radius of A11
  measures "d237" radius of A12
  measures "d238" radius of A13
  measures "d239" radius of A14
  measures "d240" radius of A15
  measures "d241" radius of A16
  measures "d242" radius of A17
  measures "d243" radius of A18
  measures "d244" radius of A19
sketch "Right-Bottom" plane through (0, 0, 0) normal (0, 0, 1) x (1, 0, 0)
  line L0 (242, 0) -> (39.975, 0)
  line L1 (250, 8) -> (250, 135.062)
  line L2 (242, 143.062) -> (39.975, 143.062)
  line L3 (242.25, 3.75) -> (37.975, 3.75)
  line L4 (246.25, 7.75) -> (246.25, 135.312)
  line L5 (242.25, 139.312) -> (37.975, 139.312)
  line L6 (37.975, 2) -> (37.975, 3.75)
  line L7 (37.975, 141.062) -> (37.975, 139.312)
  arc A0 (37.975, 2) -> (39.975, 0) centre (39.975, 2) ccw
  arc A1 (39.975, 143.062) -> (37.975, 141.062) centre (39.975, 141.062) ccw
  arc A2 (250, 135.062) -> (242, 143.062) centre (242, 135.062) ccw
  arc A3 (246.25, 135.312) -> (242.25, 139.312) centre (242.25, 135.312) ccw
  arc A4 (242, 0) -> (250, 8) centre (242, 8) ccw
  arc A5 (242.25, 3.75) -> (246.25, 7.75) centre (242.25, 7.75) ccw
  line L8 (37.975, 3.75) -> (37.975, 12)
  line L9 (37.975, 12) -> (41.975, 12)
  line L10 (45.975, 8) -> (45.975, 3.75)
  arc A6 (45.975, 8) -> (41.975, 12) centre (41.975, 8) ccw
  line L11 (136.988, 8) -> (136.988, 3.75)
  line L12 (144.988, 8) -> (144.988, 3.75)
  arc A7 (140.988, 12) -> (136.988, 8) centre (140.988, 8) ccw
  arc A8 (144.988, 8) -> (140.988, 12) centre (140.988, 8) ccw
  line L13 (238, 8) -> (238, 3.75)
  line L14 (242, 12) -> (246.25, 12)
  arc A9 (242, 12) -> (238, 8) centre (242, 8) ccw
  line L15 (238, 135.062) -> (238, 139.312)
  line L16 (242, 131.062) -> (246.25, 131.062)
  arc A10 (238, 135.062) -> (242, 131.062) centre (242, 135.062) ccw
  line L17 (37.975, 139.312) -> (37.975, 131.062)
  line L18 (37.975, 131.062) -> (41.975, 131.062)
  line L19 (45.975, 135.062) -> (45.975, 139.312)
  arc A11 (41.975, 131.062) -> (45.975, 135.062) centre (41.975, 135.062) ccw
  line L20 (66.837, 139.312) -> (66.837, 135.062)
  line L21 (70.837, 131.062) -> (90.837, 131.062)
  line L22 (94.837, 135.062) -> (94.837, 139.312)
  arc A12 (66.837, 135.062) -> (70.837, 131.062) centre (70.837, 135.062) ccw
  arc A13 (90.837, 131.062) -> (94.837, 135.062) centre (90.837, 135.062) ccw
  line L23 (185.325, 139.312) -> (185.325, 135.062)
  line L24 (181.325, 131.062) -> (161.325, 131.062)
  line L25 (157.325, 135.062) -> (157.325, 139.312)
  arc A14 (181.325, 131.062) -> (185.325, 135.062) centre (181.325, 135.062) ccw
  arc A15 (157.325, 135.062) -> (161.325, 131.062) centre (161.325, 135.062) ccw
  point P0 (250, 0)
  point P1 (37.975, 0)
  point P2 (250, 143.062)
  point P3 (37.975, 143.062)
  point P4 (45.975, 12)
  point P5 (136.988, 12)
  point P6 (144.988, 12)
  point P7 (238, 12)
  point P8 (45.975, 131.062)
  point P9 (66.837, 131.062)
  point P10 (94.837, 131.062)
  point P11 (185.325, 131.062)
  point P12 (157.325, 131.062)
  dimension "d223" = 212.025
  dimension "d224" = 143.062
  dimension "d225" = 212.025
  dimension "d245" = 2
  dimension "d246" = 2
  dimension "d247" = 8
  dimension "d248" = 4
  dimension "d249" = 8
  dimension "d250" = 4
  dimension "d251" = 8.25
  dimension "d252" = 8
  dimension "d253" = 8.25
  dimension "d254" = 4
  dimension "d255" = 99.013
  dimension "d256" = 8
  dimension "d257" = 8.25
  dimension "d258" = 4
  dimension "d259" = 4
  dimension "d262" = 8.25
  dimension "d263" = 4
  dimension "d266" = 4
  dimension "d267" = 8.25
  dimension "d268" = 8
  dimension "d269" = 4
  dimension "d270" = 20.862
  dimension "d271" = 8.25
  dimension "d272" = 28
  dimension "d273" = 4
  dimension "d274" = 4
  dimension "d275" = 52.675
  dimension "d276" = 8.25
  dimension "d277" = 28
  dimension "d278" = 4
  dimension "d279" = 4
  constraint horizontal L0
  constraint perpendicular L0 L1
  constraint perpendicular L1 L2
  constraint coincident P1 L0
  constraint coincident P1 L6
  constraint tangent L0 A0
  constraint tangent L6 A0
  constraint coincident P3 L2
  constraint coincident P3 L7
  constraint tangent L2 A1
  constraint tangent L7 A1
  constraint coincident P2 L1
  constraint coincident P2 L2
  constraint tangent L1 A2
  constraint tangent L2 A2
  constraint tangent L4 A3
  constraint tangent L5 A3
  constraint coincident P0 L0
  constraint coincident P0 L1
  constraint tangent L0 A4
  constraint tangent L1 A4
  constraint tangent L3 A5
  constraint tangent L4 A5
  constraint perpendicular L3 L8
  constraint perpendicular L8 L9
  constraint perpendicular L3 L10
  constraint coincident P4 L9
  constraint coincident P4 L10
  constraint tangent L9 A6
  constraint tangent L10 A6
  constraint coincident L3 L11.end
  constraint perpendicular L3 L11
  constraint coincident P5 L11
  constraint tangent L11 A7
  constraint coincident P6 L12
  constraint tangent L12 A8
  constraint coincident A7.start A8.end
  constraint perpendicular L3 L13
  constraint coincident L4 L14.end
  constraint perpendicular L4 L14
  constraint coincident P7 L13
  constraint coincident P7 L14
  constraint tangent L13 A9
  constraint tangent L14 A9
  constraint coincident L5 L15.end
  constraint perpendicular L5 L15
  constraint coincident L4 L16.end
  constraint perpendicular L4 L16
  constraint tangent L15 A10
  constraint tangent L16 A10
  constraint perpendicular L5 L17
  constraint perpendicular L17 L18
  constraint coincident L5 L19.end
  constraint perpendicular L5 L19
  constraint coincident P8 L18
  constraint coincident P8 L19
  constraint tangent L18 A11
  constraint tangent L19 A11
  constraint perpendicular L5 L20
  constraint perpendicular L20 L21
  constraint coincident L5 L22.end
  constraint perpendicular L5 L22
  constraint coincident P9 L20
  constraint coincident P9 L21
  constraint tangent L20 A12
  constraint tangent L21 A12
  constraint coincident P10 L21
  constraint coincident P10 L22
  constraint tangent L21 A13
  constraint tangent L22 A13
  constraint perpendicular L5 L23
  constraint perpendicular L23 L24
  constraint coincident L5 L25.end
  constraint perpendicular L5 L25
  constraint coincident P11 L23
  constraint coincident P11 L24
  constraint tangent L23 A14
  constraint tangent L24 A14
  constraint coincident P12 L24
  constraint coincident P12 L25
  constraint tangent L24 A15
  constraint tangent L25 A15
  measures "d223" distance of P0 P1
  measures "d224" distance of P0 P2
  measures "d225" distance of P2 P3
  measures "d245" radius of A0
  measures "d246" radius of A1
  measures "d247" radius of A2
  measures "d248" radius of A3
  measures "d249" radius of A4
  measures "d250" radius of A5
  measures "d251" distance of L3.end L8.end
  measures "d252" distance of L8.end P4
  measures "d253" distance of P4 L10.end
  measures "d254" radius of A6
  measures "d255" distance of L8.end P5
  measures "d256" distance of P5 P6
  measures "d257" distance of P6 L12.end
  measures "d258" radius of A7
  measures "d259" radius of A8
  measures "d262" distance of P7 L13.end
  measures "d263" radius of A9
  measures "d266" radius of A10
  measures "d267" distance of L5.end L17.end
  measures "d268" distance of L17.end P8
  measures "d269" radius of A11
  measures "d270" distance of L19.end L20.start
  measures "d271" distance of L20.start P9
  measures "d272" distance of P9 P10
  measures "d273" radius of A12
  measures "d274" radius of A13
  measures "d275" distance of L15.end L23.start
  measures "d276" distance of L23.start P11
  measures "d277" distance of P11 P12
  measures "d278" radius of A14
  measures "d279" radius of A15
sketch "Right-USB" plane through (0, 0, 0) normal (0, 1, 0) x (1, 0, 0)
  line L0 (77.8375, -8) -> (83.8375, -8)
  arc A0 (83.8375, -8) -> (83.8375, -4.2) centre (83.8375, -6.1) ccw
  line L1 (83.8375, -4.2) -> (77.8375, -4.2)
  arc A1 (77.8375, -4.2) -> (77.8375, -8) centre (77.8375, -6.1) ccw
  line L2 (77.8375, -6.1) -> (83.8375, -6.1) construction
  line L3 (77.8375, -10) -> (83.8375, -10)
  arc A2 (83.8375, -10) -> (83.8375, -2.2) centre (83.8375, -6.1) ccw
  line L4 (83.8375, -2.2) -> (77.8375, -2.2)
  arc A3 (77.8375, -2.2) -> (77.8375, -10) centre (77.8375, -6.1) ccw
  line L5 (77.8375, -6.1) -> (83.8375, -6.1) construction
  line L6 (168.325, -8) -> (174.325, -8)
  arc A4 (174.325, -8) -> (174.325, -4.2) centre (174.325, -6.1) ccw
  line L7 (174.325, -4.2) -> (168.325, -4.2)
  arc A5 (168.325, -4.2) -> (168.325, -8) centre (168.325, -6.1) ccw
  line L8 (168.325, -6.1) -> (174.325, -6.1) construction
  line L9 (168.325, -10) -> (174.325, -10)
  arc A6 (174.325, -10) -> (174.325, -2.2) centre (174.325, -6.1) ccw
  line L10 (174.325, -2.2) -> (168.325, -2.2)
  arc A7 (168.325, -2.2) -> (168.325, -10) centre (168.325, -6.1) ccw
  line L11 (168.325, -6.1) -> (174.325, -6.1) construction
  line L12 (168.325, -6.1) -> (166.425, -6.1)
  line L13 (166.425, -6.1) -> (166.425, -7.4)
  line L14 (165.775, -8.05) -> (165.775, -11.3)
  line L15 (165.775, -11.3) -> (176.875, -11.3)
  line L16 (176.875, -11.3) -> (176.875, -8.05)
  line L17 (174.325, -6.1) -> (176.225, -6.1)
  line L18 (176.225, -6.1) -> (176.225, -7.4)
  line L19 (83.8375, -6.1) -> (85.7375, -6.1)
  line L20 (77.8375, -6.1) -> (75.9375, -6.1)
  line L21 (75.9375, -6.1) -> (75.9375, -7.4)
  line L22 (75.2875, -8.05) -> (75.2875, -11.3)
  line L23 (75.2875, -11.3) -> (86.3875, -11.3)
  line L24 (86.3875, -11.3) -> (86.3875, -8.05)
  line L25 (85.7375, -6.1) -> (85.7375, -7.4)
  arc A8 (75.9375, -7.4) -> (75.2875, -8.05) centre (75.9375, -8.05) ccw
  arc A9 (86.3875, -8.05) -> (85.7375, -7.4) centre (85.7375, -8.05) ccw
  arc A10 (166.425, -7.4) -> (165.775, -8.05) centre (166.425, -8.05) ccw
  arc A11 (176.875, -8.05) -> (176.225, -7.4) centre (176.225, -8.05) ccw
  point P0 (165.775, -7.4)
  point P1 (75.2875, -7.4)
  dimension "d280" = 0.65
  dimension "d281" = 11.1
  dimension "d282" = 0.65
  dimension "d283" = 11.1
  dimension "d284" = 0.65
  dimension "d285" = 0.65
  dimension "d286" = 0.65
  dimension "d287" = 0.65
  constraint tangent L0 A0
  constraint tangent A0 L1
  constraint parallel L0 L1
  constraint tangent L1 A1
  constraint tangent L0 A1
  constraint horizontal L2
  constraint tangent L3 A2
  constraint tangent A2 L4
  constraint parallel L3 L4
  constraint tangent L4 A3
  constraint tangent L3 A3
  constraint coincident A0.centre L2.end
  constraint parallel L2 L5
  constraint coincident A1.centre L2.start
  constraint tangent L6 A4
  constraint tangent A4 L7
  constraint parallel L6 L7
  constraint tangent L7 A5
  constraint tangent L6 A5
  constraint horizontal L8
  constraint tangent L9 A6
  constraint tangent A6 L10
  constraint parallel L9 L10
  constraint tangent L10 A7
  constraint tangent L9 A7
  constraint coincident A4.centre L8.end
  constraint parallel L8 L11
  constraint coincident A5.centre L8.start
  constraint midpoint A5 L12.end
  constraint tangent A5 L13
  constraint perpendicular L12 L13
  constraint perpendicular L14 L15
  constraint perpendicular L15 L16
  constraint midpoint A4 L17.end
  constraint tangent A4 L18
  constraint perpendicular L17 L18
  constraint midpoint A0 L19.end
  constraint midpoint A1 L20.end
  constraint tangent A1 L21
  constraint perpendicular L20 L21
  constraint perpendicular L22 L23
  constraint perpendicular L3 L24
  constraint tangent A0 L25
  constraint perpendicular L19 L25
  constraint coincident P1 L22
  constraint tangent L22 A8
  constraint coincident L21.end A8.start
  constraint tangent L24 A9
  constraint coincident L25.end A9.end
  constraint coincident P0 L14
  constraint tangent L14 A10
  constraint coincident L13.end A10.start
  constraint tangent L16 A11
  constraint coincident L18.end A11.end
  measures "d280" distance of L13.end P0
  measures "d281" distance of L14.end L15.end
  measures "d282" distance of L21.end P1
  measures "d283" distance of L22.end L23.end
  measures "d284" radius of A8
  measures "d285" radius of A9
  measures "d286" radius of A10
  measures "d287" radius of A11